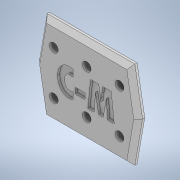
# Autodesk Inventor part: front brackets magnet
Saved by Autodesk Inventor 2022 (Build 260153000, 153)
## iProperties
Created: 2023-03-09
Part Number: front brackets magnet
Material: Generic
Document SubType Name: Modeling
Designer: chris
Density: 1 g/cm^3
Appearance: Default
Author: chris
Autodesk Inventor part; units mm, degrees
ref_plane "YZ Plane" through (0, 0, 0) normal (1, 0, 0) x (0, 1, 0)
ref_plane "XZ Plane" through (0, 0, 0) normal (0, 1, 0) x (-1, 0, 0)
ref_plane "XY Plane" through (0, 0, 0) normal (0, 0, 1) x (1, 0, 0)
sketch "Sketch1" plane through (0, 0, 0) normal (0, 0, 1) x (1, 0, 0)
  line L0 (0, 0) -> (0, -10)
  line L1 (0, -10) -> (15, -10)
  line L2 (15, -10) -> (-15, -10)
  circle A0 centre (0, -10) radius 2
  circle A1 centre (-15, -10) radius 2
  circle A2 centre (15, -10) radius 2
  circle A3 centre (15, 10) radius 2
  line L3 (0, 10) -> (15, 10)
  line L4 (0, 0) -> (0, 10)
  circle A4 centre (0, 10) radius 2
  line L5 (15, 10) -> (-15, 10)
  circle A5 centre (-15, 10) radius 2
  line L6 (0, 20) -> (-20, 20)
  line L7 (0, -20) -> (-20, -20)
  line L8 (0, 20) -> (20, 20)
  line L9 (0, -20) -> (20, -20)
  line L10 (-9.0875, 18.9456) -> (0.4518, 18.9456) construction
  line L11 (0.4518, 18.9456) -> (0.4518, 15.7414) construction
  line L12 (0.4518, 15.7414) -> (-9.0875, 15.7414) construction
  line L13 (-9.0875, 15.7414) -> (-9.0875, 18.9456) construction
  line L14 (-14.2732, -12.6124) -> (-4.734, -12.6124) construction
  line L15 (-4.734, -12.6124) -> (-4.734, -15.8166) construction
  line L16 (-4.734, -15.8166) -> (-14.2732, -15.8166) construction
  line L17 (-14.2732, -15.8166) -> (-14.2732, -12.6124) construction
  line L18 (0, 0) -> (-23.5, 0)
  line L19 (-23.5, 0) -> (-20, 20)
  line L20 (0, 0) -> (23.5, 0)
  line L21 (23.5, 0) -> (20, 20)
  line L22 (-23.5, 0) -> (-20, -20)
  line L23 (23.5, 0) -> (20, -20)
  point P0 (0, 0)
  point P1 (0, 0)
  point P2 (0, 0)
  point P3 (0, 0)
  dimension "d0" = 10
  dimension "d1" = 15
  dimension "d2" = 30
  dimension "d3" = 4
  dimension "d4" = 4
  dimension "d5" = 4
  dimension "d7" = 20
  dimension "d24" = 23.5
  dimension "d25" = 23.5
  constraints: 32 end point, 7 coincident, 6 centre point, 2 point on line, 1 horizontal, 1 midpoint, 1 perpendicular, 4 other
  measures "d0" distance of L0.start L1.start
  measures "d1" distance of L1.start L1.end
  measures "d2" distance of L1.end L2.end
  measures "d3" diameter of A0
  measures "d4" diameter of A1
  measures "d5" diameter of A2
  measures "d7" distance of L6.start L6.end
  measures "d24" distance of L0.start L18.end
  measures "d25" distance of L0.start L20.end
extrude "Extrusion1" add sketch "Sketch1" along normal blind 3
sketch "Sketch2" plane through (0, 0, 3) normal (0, 0, 1) x (1, 0, 0)
  line L0 (0, 20) -> (-20, 20)
  line L1 (-20, 20) -> (-25.359, 0)
  line L2 (-20, -20) -> (-25.359, 0)
  line L3 (0, -20) -> (-20, -20)
  line L4 (0, 20) -> (20, 20)
  line L5 (20, 20) -> (25.359, 0)
  line L6 (20, -20) -> (25.359, 0)
  line L7 (0, -20) -> (20, -20)
  line L8 (-13.9831, 6.124) -> (-4.4439, 6.124) construction
  line L9 (-4.4439, 6.124) -> (-4.4439, 2.9198) construction
  line L10 (-4.4439, 2.9198) -> (-13.9831, 2.9198) construction
  line L11 (-13.9831, 2.9198) -> (-13.9831, 6.124) construction
  line L12 (-6.2592, -3.0831) -> (-6.2592, -6.1649)
  spline S0 degree 2 poles (-6.2592, -6.1649) (-7.2511, -6.4828) (-7.9446, -6.4828) knots 0 0 0 1 1 1
  spline S1 degree 2 poles (-7.9446, -6.4828) (-10.3234, -6.4828) (-13.2704, -2.9194) (-13.2704, -0.0494) knots 0 0 0 1 2 2 2
  spline S2 degree 2 poles (-13.2704, -0.0494) (-13.2704, 2.6184) (-10.2945, 6.124) (-8.012, 6.124) knots 0 0 0 1 2 2 2
  spline S3 degree 2 poles (-8.012, 6.124) (-7.1259, 6.124) (-6.2592, 5.8447) knots 0 0 0 1 1 1
  line L13 (-6.2592, 5.8447) -> (-6.2592, 2.7725)
  spline S4 degree 2 poles (-6.2592, 2.7725) (-7.2319, 3.0229) (-7.8675, 3.0229) knots 0 0 0 1 1 1
  spline S5 degree 2 poles (-7.8675, 3.0229) (-8.8113, 3.0229) (-10.073, 1.2604) (-10.073, -0.1361) knots 0 0 0 1 2 2 2
  spline S6 degree 2 poles (-10.073, -0.1361) (-10.073, -1.6481) (-8.8017, -3.3527) (-7.7519, -3.3527) knots 0 0 0 1 2 2 2
  spline S7 degree 2 poles (-7.7519, -3.3527) (-7.2222, -3.3527) (-6.2592, -3.0831) knots 0 0 0 1 1 1
  line L14 (-5.1227, -0.7428) -> (-0.7407, -0.7428)
  line L15 (-0.7407, -0.7428) -> (-0.7407, -3.2853)
  line L16 (-0.7407, -3.2853) -> (-5.1227, -3.2853)
  line L17 (-5.1227, -3.2853) -> (-5.1227, -0.7428)
  line L18 (1.8211, 5.8062) -> (5.4808, 5.8062)
  spline S8 degree 2 poles (5.4808, 5.8062) (6.2224, 1.8383) (6.4535, -0.6657) knots 0 0 0 1 1 1
  line L19 (6.4535, -0.6657) -> (6.5595, 0.9811)
  spline S9 degree 2 poles (6.5595, 0.9811) (6.7328, 1.9827) (6.9351, 3.0421) knots 0 0 0 1 1 1
  line L20 (6.9351, 3.0421) -> (7.4744, 5.8062)
  line L21 (7.4744, 5.8062) -> (11.2015, 5.8062)
  line L22 (11.2015, 5.8062) -> (12.5498, -6.1938)
  line L23 (12.5498, -6.1938) -> (9.5739, -6.1938)
  line L24 (9.5739, -6.1938) -> (8.9672, 1.8094)
  line L25 (8.9672, 1.8094) -> (7.5611, -6.1938)
  line L26 (7.5611, -6.1938) -> (5.4712, -6.1938)
  line L27 (5.4712, -6.1938) -> (3.988, 1.8286)
  line L28 (3.988, 1.8286) -> (3.4005, -6.1938)
  line L29 (3.4005, -6.1938) -> (0.5498, -6.1938)
  line L30 (0.5498, -6.1938) -> (1.8211, 5.8062)
  dimension "d20" = 20
  dimension "d21" = 105
  constraints: 16 end point, 2 other
  measures "d20" distance of L4.start L1.start
  measures "d21" angle of L1 L0
chamfer "Chamfer1" distance 2 angle 45 4 edges at (-10, 20, 3) (10, 20, 3) (-10, -20, 3) (10, -20, 3)
extrude "Extrusion2" cut sketch "Sketch2" against normal blind 1 contours L12 S0 S1 S2 S3 L13 S4 S5 S6 S7 | L14 L15 L16 L17 | L18 S8 L19 S9 L20 L21 L22 L23 L24 L25 L26 L27 L28 L29 L30
chamfer "Chamfer2" distance 2 angle 45 4 edges at (-21.925, 9, 3) (-21.925, -9, 3) (21.925, 9, 3) (21.925, -9, 3)
body "Solid1"
